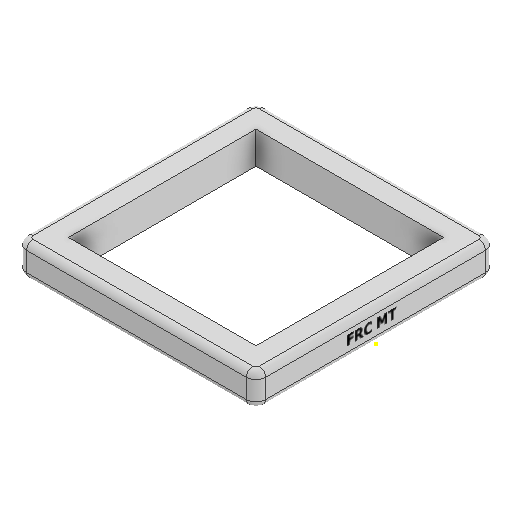
# Autodesk Inventor part: Bumper
Saved by Autodesk Inventor 2025.3 (Build 293356000, 356)
## iProperties
Created: 2026-05-15
Part Number: Bumper
Material: Genérico
Document SubType Name: Modeling
Designer: djair.oliveira
Density: 1 g/cm^3
Appearance: Padrão
Author: djair.oliveira
Autodesk Inventor part; units mm, degrees
ref_plane "YZ Plane" through (0, 0, 0) normal (1, 0, 0) x (0, 1, 0)
ref_plane "XZ Plane" through (0, 0, 0) normal (0, 1, 0) x (-1, 0, 0)
ref_plane "XY Plane" through (0, 0, 0) normal (0, 0, 1) x (1, 0, 0)
sketch "Esboço1" plane through (0, 0, 0) normal (0, 1, 0) x (-1, 0, 0)
  line L0 (-292.1, 292.1) -> (292.1, 292.1)
  line L1 (292.1, 292.1) -> (292.1, -292.1)
  line L2 (292.1, -292.1) -> (-292.1, -292.1)
  line L3 (-292.1, -292.1) -> (-292.1, 292.1)
  line L4 (-292.1, 292.1) -> (292.1, -292.1) construction
  line L5 (292.1, 292.1) -> (-292.1, -292.1) construction
  line L6 (-342.1, 372.1) -> (342.1, 372.1)
  line L7 (372.1, 342.1) -> (372.1, -342.1)
  line L8 (342.1, -372.1) -> (-342.1, -372.1)
  line L9 (-372.1, -342.1) -> (-372.1, 342.1)
  line L10 (-372.1, 372.1) -> (372.1, -372.1) construction
  line L11 (372.1, 372.1) -> (-372.1, -372.1) construction
  arc A0 (-372.1, -342.1) -> (-342.1, -372.1) centre (-342.1, -342.1) ccw
  arc A1 (-342.1, 372.1) -> (-372.1, 342.1) centre (-342.1, 342.1) ccw
  arc A2 (372.1, 342.1) -> (342.1, 372.1) centre (342.1, 342.1) ccw
  arc A3 (342.1, -372.1) -> (372.1, -342.1) centre (342.1, -342.1) ccw
  point P0 (0, 0)
  dimension "d0" = 584.2
  dimension "d1" = 584.2
  dimension "d2" = 80
  dimension "d3" = 30
  constraints: 24 end point, 9 point on line, 8 point on circle, 8 tangent, 4 centre point, 4 midpoint, 4 parallel, 3 equal radius, 2 horizontal, 2 perpendicular
  measures "d0" distance of L0.end L1.end
  measures "d1" distance of L1.end L2.end
  measures "d2" distance between parallel lines of L9 L3
  measures "d3" radius of A0
extrude "Extrusão1" add sketch "Esboço1" along normal blind 100
fillet "Arredondamento1" radius 20 16 edges at (363.3132, 100, -363.3132) (0, 100, -372.1) (-363.3132, 100, -363.3132) (-372.1, 100, 0) (-363.3132, 100, 363.3132) (0, 100, 372.1) (363.3132, 100, 363.3132) (372.1, 100, 0) (363.3132, 0, -363.3132) (0, 0, -372.1) (-363.3132, 0, -363.3132) (-372.1, 0, 0) (-363.3132, 0, 363.3132) (0, 0, 372.1) (363.3132, 0, 363.3132) (372.1, 0, 0)
sketch "Esboço2" plane through (372.1, 20, -342.1) normal (1, 0, 0) x (0, 0, -1)
  line L0 (-443.4891, 47.2081) -> (-266.8261, 47.2081) construction
  line L1 (-266.8261, 47.2081) -> (-266.8261, 12.6629) construction
  line L2 (-266.8261, 12.6629) -> (-443.4891, 12.6629) construction
  line L3 (-443.4891, 12.6629) -> (-443.4891, 47.2081) construction
  point P0 (-342.1, -20)
  constraints: 2 other
equation "\"d1\" = d0"
